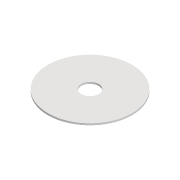
# Autodesk Inventor part: 垃圾桶
Saved by Autodesk Inventor 2021 (Build 250183000, 183)
## iProperties
Created: 2025-04-17
Part Number: 垃圾桶
Material: 常规
Document SubType Name: Modeling
Designer: 86155
Density: 1 g/cm^3
Appearance: 默认
Author: 86155
Autodesk Inventor part; units mm, degrees
ref_plane "YZ Plane" through (0, 0, 0) normal (1, 0, 0) x (0, 1, 0)
ref_plane "XZ Plane" through (0, 0, 0) normal (0, 1, 0) x (-1, 0, 0)
ref_plane "XY Plane" through (0, 0, 0) normal (0, 0, 1) x (1, 0, 0)
sketch "草图1" plane through (0, 0, 0) normal (0, 1, 0) x (-1, 0, 0)
  circle A0 centre (0, 0) radius 50
  circle A1 centre (0, 0) radius 240
  dimension "d0" = 100
  dimension "d1" = 480
  constraints: 2 centre point, 2 coincident
  measures "d0" diameter of A0
  measures "d1" diameter of A1
extrude "拉伸1" add sketch "草图1" along normal blind 10
sketch "草图2" plane through (0, 10, 0) normal (0, 1, 0) x (1, 0, 0)
  line L0 (32.8343, 37.7082) -> (142.765, 192.92) projected
  arc A0 (48.9841, -10.0277) -> (32.8343, 37.7082) centre (0, 0) ccw projected
  line L1 (230.5699, -66.6149) -> (48.9841, -10.0277) projected
  circle A1 centre (0, 0) radius 240 projected
extrude "拉伸2" add sketch "草图2" along normal blind 380 contours L0 A1 L1 A0 picked at (176.373, 6.3513)
sketch "草图3" plane through (0, 10, 0) normal (0, 1, 0) x (1, 0, 0)
  line L0 (32.8343, 37.7082) -> (142.765, 192.92) projected
  arc A0 (142.765, 192.92) -> (230.5699, -66.6149) centre (0, 0) ccw projected
  line L1 (230.5699, -66.6149) -> (48.9841, -10.0277) projected
  arc A1 (32.8343, 37.7082) -> (48.9841, -10.0277) centre (0, 0) ccw projected
extrude "拉伸3" cut sketch "草图3" against normal blind 10
sketch "草图4" plane through (0, 390, 0) normal (0, 1, 0) x (1, 0, 0)
  circle A0 centre (0, 0) radius 50
  circle A1 centre (0, 0) radius 40
  line L0 (48.9841, -10.0277) -> (230.5699, -66.6149) projected
  line L1 (0, 0) -> (48.9841, -10.0277)
  line L2 (142.765, 192.92) -> (32.8343, 37.7082) projected
  line L3 (0, 0) -> (32.8343, 37.7082)
  point P0 (26.2675, 30.1665)
  point P1 (39.1873, -8.0221)
  dimension "d8" = 80
  constraints: 4 end point, 2 centre point, 2 coincident
  measures "d8" diameter of A1
extrude "拉伸4" add sketch "草图4" against normal blind 350 contours A0 L1 A1 L3 picked at (37.3478, 21.6697)
sketch "草图5" plane through (0, 390, 0) normal (0, 1, 0) x (1, 0, 0)
  line L0 (48.9841, -10.0277) -> (230.5699, -66.6149) projected
  arc A0 (230.5699, -66.6149) -> (142.765, 192.92) centre (0, 0) ccw projected
  line L1 (142.765, 192.92) -> (32.8343, 37.7082) projected
  line L2 (32.8343, 37.7082) -> (26.2675, 30.1665) projected
  arc A1 (39.1873, -8.0221) -> (26.2675, 30.1665) centre (0, 0) ccw projected
  line L3 (39.1873, -8.0221) -> (48.9841, -10.0277) projected
  line L4 (38.7374, 33.0665) -> (144.3863, 182.2329)
  arc A2 (225.3695, -57.1386) -> (144.3863, 182.2329) centre (0, 0) ccw
  line L5 (225.3695, -57.1386) -> (50.8566, -2.7555)
  line L6 (50.8566, -2.7555) -> (47.4553, -2.0592)
  arc A3 (47.4553, -2.0592) -> (36.4576, 30.4483) centre (0, 0) ccw
  line L7 (36.4576, 30.4483) -> (38.7374, 33.0665)
  dimension "d11" = 7.5
  constraints: 8 end point, 4 point on circle, 2 centre point, 5 other
  measures "d11" distance between parallel lines of L1 L4
extrude "拉伸5" cut sketch "草图5" against normal blind 340 contours L4 A2 L5 L6 A3 L7
